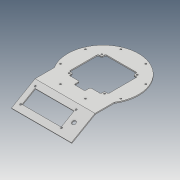
# Autodesk Inventor part: 모터드라이버 지지대 철판가공
Saved by Autodesk Inventor 2018 (Build 220112000, 112)
## iProperties
Created: 2018-10-26
Part Number: 모터드라이버 지지대 철판가공
Material: 일반
Document SubType Name: Modeling
Designer: dhksr
Density: 1 g/cm^3
Appearance: 기본값
Author: dhksr
Autodesk Inventor part; units mm, degrees
ref_plane "YZ Plane" through (0, 0, 0) normal (1, 0, 0) x (0, 1, 0)
ref_plane "XZ Plane" through (0, 0, 0) normal (0, 1, 0) x (-1, 0, 0)
sketch "스케치1" plane through (0, 0, 0) normal (0, 0, 1) x (1, 0, 0)
  circle A0 centre (0, 0) radius 60 construction
  circle A1 centre (0, 0) radius 65
  circle A2 centre (-60, 0) radius 1.5
  line L0 (-36, 0) -> (-36, 26.5)
  line L1 (-36, 26.5) -> (-29, 26.5)
  line L2 (-29, 26.5) -> (-29, 33.5)
  line L3 (-29, 33.5) -> (0, 33.5)
  line L4 (0, 0) -> (0, 95.3997)
  line L5 (0, 0) -> (-132.5472, 0)
  circle A3 centre (-32.5, 30) radius 1.5
  line L6 (36, 0) -> (36, 26.5)
  line L7 (36, 26.5) -> (29, 26.5)
  line L8 (29, 26.5) -> (29, 33.5)
  line L9 (29, 33.5) -> (0, 33.5)
  circle A4 centre (32.5, 30) radius 1.5
  line L10 (-36, 0) -> (-36, -26.5)
  line L11 (-36, -26.5) -> (-29, -26.5)
  line L12 (-29, -26.5) -> (-29, -33.5)
  line L13 (-29, -33.5) -> (0, -33.5)
  circle A5 centre (-32.5, -30) radius 1.5
  line L14 (36, 0) -> (36, -26.5)
  line L15 (36, -26.5) -> (29, -26.5)
  line L16 (29, -26.5) -> (29, -33.5)
  line L17 (29, -33.5) -> (0, -33.5)
  circle A6 centre (32.5, -30) radius 1.5
  point P0 (-29, 30)
  point P1 (-32.5, 26.5)
  point P2 (29, 30)
  point P3 (32.5, 26.5)
  point P4 (-29, -30)
  point P5 (-32.5, -26.5)
  point P6 (29, -30)
  point P7 (32.5, -26.5)
  dimension "d0" = 120
  dimension "d1" = 130
  dimension "d2" = 3
  dimension "d3" = 3
  dimension "d4" = 65
  dimension "d6" = 60
  dimension "d9" = 72
  dimension "d10" = 67
  constraints: 36 end point, 20 symmetric about line, 6 centre point, 5 coincident, 3 horizontal alignment, 3 perpendicular, 2 midpoint, 2 vertical, 2 vertical alignment, 1 horizontal, 5 other
  measures "d1" diameter of A1
  measures "d2" diameter of A2
  measures "d3" diameter of A3
  measures "d4" diameter of A3.centre L4
  measures "d6" diameter of A3.centre L5
  measures "d9" distance between parallel lines of L6 L0
  measures "d10" distance between parallel lines of L17 L9
extrude "돌출1" add sketch "스케치1" along normal blind 2 contours A1 L5 A2 L10 L11 L12 L13 L17 L16 L15 L14 L6 L7 L8 L9 L4 | L4 L3 L2 L1 L0 L5 A2 A1 | L5 A2 | A2 L5
fillet "모깎기1" radius 2 3 edges at (-36, 26.5, 1) (-29, 26.5, 1) (-29, 33.5, 1)
mirror "미러1" about plane through (0, 0, 0) normal (1, 0, 0) of "모깎기1"
mirror "미러2" about plane through (0, 0, 0) normal (0, 1, 0) of "모깎기1", "미러1"
sketch "스케치3" plane through (0, 0, 2) normal (0, 0, 1) x (1, 0, 0)
  line L0 (10, -23.5) -> (-10, -23.5)
  line L1 (-10, -23.5) -> (-10, -43.5)
  line L2 (-10, -43.5) -> (10, -43.5)
  line L3 (10, -43.5) -> (10, -23.5)
  line L4 (10, -23.5) -> (-10, -43.5) construction
  line L5 (-10, -23.5) -> (10, -43.5) construction
  point P0 (0, -33.5)
  dimension "d25" = 20
  dimension "d26" = 20
  constraints: 12 end point, 2 midpoint, 2 parallel, 1 horizontal, 1 perpendicular
  measures "d25" distance of L2.end L1.end
  measures "d26" distance of L1.end L0.end
extrude "돌출3" cut sketch "스케치3" against normal through all
fillet "모깎기2" radius 2 4 edges at (-10, -33.5, 1) (-10, -43.5, 1) (10, -43.5, 1) (10, -33.5, 1)
sketch "스케치4" plane through (0, 0, 2) normal (0, 0, 1) x (1, 0, 0)
  circle A0 centre (0, 0) radius 60 construction
  line L0 (0, 0) -> (87.146, 36.0971) construction
  line L1 (0, 0) -> (94.3262, 0) construction
  circle A1 centre (55.4328, 22.961) radius 1.5
  dimension "d28" = 120
  dimension "d29" = 22.5
  dimension "d30" = 3
  constraints: 4 end point, 1 centre point, 1 coincident, 1 equal length, 1 horizontal, 1 point on line, 3 other
  measures "d29" angle of L1 L0
  measures "d30" diameter of A1
extrude "돌출4" cut sketch "스케치4" against normal through all
pattern_circular "원형 패턴1" count 8 over 360 about axis through (0, 0, 0) along (0, 0, 1) of "돌출4"
sketch "스케치7" plane through (0, 0, 2) normal (0, 0, 1) x (1, 0, 0)
  circle A0 centre (22.961, -55.4328) radius 1.5 projected
  circle A1 centre (-22.961, -55.4328) radius 1.5 projected
  line L0 (10, -35.5) -> (10, -41.5) projected
  arc A2 (8, -43.5) -> (10, -41.5) centre (8, -41.5) ccw projected
  line L1 (8, -43.5) -> (-8, -43.5) projected
  arc A3 (-10, -41.5) -> (-8, -43.5) centre (-8, -41.5) ccw projected
  line L2 (-10, -41.5) -> (-10, -35.5) projected
  line L3 (55, -70) -> (-55, -70)
  line L4 (-55, -70) -> (-55, -38.5)
  line L5 (55, -38.5) -> (55, -70)
  line L6 (55, -70) -> (-55, -38.5) construction
  line L7 (-55, -70) -> (55, -38.5) construction
  circle A4 centre (0, 0) radius 65 projected
  line L8 (-55, -38.5) -> (-55, -30)
  line L9 (-55, -30) -> (-25.3175, -38.5)
  line L10 (55, -38.5) -> (55, -27.7769)
  line L11 (55, -27.7769) -> (39.506, -38.5)
  line L12 (10, -38.5) -> (39.506, -38.5)
  line L13 (-25.3175, -38.5) -> (-10, -38.5)
  point P0 (0, -54.25)
  point P1 (0, -54.25)
  point P2 (0, -43.5)
  point P3 (-10, -38.5)
  dimension "d37" = 110
  dimension "d38" = 5
  constraints: 22 end point, 8 midpoint, 3 parallel, 2 horizontal alignment, 2 vertical, 1 horizontal, 1 perpendicular, 1 vertical alignment
  measures "d37" distance of L4.end L5.start
  measures "d38" distance edge to line of A4 L3
extrude "돌출5" add sketch "스케치7" against normal up to surface (2 mm away) contours L12 L11 L10 A4 L8 L9 L13 L2 A3 L1 A2 L0 | L10 L5 L3 L4 L8 A4 picked at (24.2159, -43.6479)
ref_plane "작업 평면3" through (55, -70, 2) normal (0, -0.5, 0.8660254) x (1, 0, 0)
sketch "스케치8" plane through (55, -70, 2) normal (0, -0.5, 0.8660254) x (1, 0, 0)
  line L0 (0, 0) -> (-110, 0) projected
  line L1 (-110, 0) -> (0, 0)
  line L2 (0, 0) -> (0, -50)
  line L3 (0, -50) -> (-110, -50)
  line L4 (-110, -50) -> (-110, 0)
  line L5 (-100.5, -38.75) -> (-28.5, -38.75)
  line L6 (-28.5, -38.75) -> (-28.5, -11.25)
  line L7 (-28.5, -11.25) -> (-100.5, -11.25)
  line L8 (-100.5, -11.25) -> (-100.5, -38.75)
  line L9 (-100.5, -38.75) -> (-28.5, -11.25) construction
  line L10 (-28.5, -38.75) -> (-100.5, -11.25) construction
  line L11 (-27.25, -8.5) -> (-102.25, -8.5) construction
  line L12 (-102.25, -8.5) -> (-102.25, -39.5) construction
  line L13 (-102.25, -39.5) -> (-27.25, -39.5) construction
  line L14 (-27.25, -39.5) -> (-27.25, -8.5) construction
  line L15 (-27.25, -8.5) -> (-102.25, -39.5) construction
  line L16 (-102.25, -8.5) -> (-27.25, -39.5) construction
  circle A0 centre (-102.25, -8.5) radius 1.5
  circle A1 centre (-102.25, -39.5) radius 1.5
  circle A2 centre (-27.25, -39.5) radius 1.5
  circle A3 centre (-27.25, -8.5) radius 1.5
  line L17 (-100.5, -25) -> (-9.5, -25)
  circle A4 centre (-17, -25) radius 3.5
  line L18 (-64.5, -11.25) -> (-64.5, -38.75)
  line L19 (-26.25, -31) -> (-7.75, -31)
  line L20 (-7.75, -31) -> (-7.75, -19)
  line L21 (-7.75, -19) -> (-26.25, -19)
  line L22 (-26.25, -19) -> (-26.25, -31)
  line L23 (-26.25, -31) -> (-7.75, -19) construction
  line L24 (-7.75, -31) -> (-26.25, -19) construction
  line L25 (-102.25, -25) -> (-7.75, -25)
  line L26 (-64.75, -24) -> (-64.5, -24)
  line L27 (-64.5, -25) -> (-64.5, -24)
  point P0 (-55, 59.6218)
  point P1 (-110, -25)
  point P2 (0, -25)
  point P3 (-55, -25)
  point P4 (-55, 0)
  point P5 (-55, -25)
  point P6 (-55, 0)
  dimension "d42" = 72
  dimension "d43" = 27.5
  dimension "d44" = 75
  dimension "d45" = 31
  dimension "d46" = 3
  dimension "d47" = 3
  dimension "d48" = 3
  dimension "d49" = 3
  dimension "d52" = 7
  dimension "d54" = 18.5
  dimension "d55" = 12
  dimension "d57" = 11.5
  dimension "d62" = 94.5
  dimension "d63" = 1
  dimension "d64" = 50
  constraints: 54 end point, 14 midpoint, 9 parallel, 5 centre point, 5 horizontal, 5 point on line, 4 coincident, 4 perpendicular, 3 vertical alignment, 2 horizontal alignment
  measures "d42" distance of L7.end L6.end
  measures "d43" distance of L6.end L5.end
  measures "d44" distance of L13.end L12.end
  measures "d45" distance of L12.end L11.end
  measures "d46" diameter of A0
  measures "d47" diameter of A1
  measures "d48" diameter of A2
  measures "d49" diameter of A3
  measures "d52" diameter of A4
  measures "d54" distance of L21.end L20.end
  measures "d55" distance of L20.end L19.end
  measures "d57" distance from line of L6 A4.centre
  measures "d62" distance of L25.start L25.end
  measures "d63" vertical distance of L26.start L27.start
  measures "d64" distance of L3.end L0.end
extrude "돌출6" add sketch "스케치8" against normal blind 2 contours L2 L3 L4 L0 | A4 L17 L22 L21 L20 L25 | L17 L25 L20 L19 L22 A4
